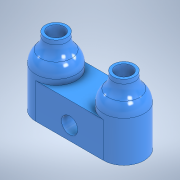
# Autodesk Inventor part: 4mm_Roller_Spacer_full
Saved by Autodesk Inventor 2021 (Build 250183000, 183)
## iProperties
Created: 2021-07-05
Part Number: 4mm_Roller_Spacer_full
Material: Generic
Document SubType Name: Modeling
Designer: Jorian Brusind
Density: 1 g/cm^3
Appearance: Cyan
Author: Jorian Brusind
Autodesk Inventor part; units mm, degrees
ref_plane "XZ Plane" through (0, 0, 0) normal (0, 1, 0) x (-1, 0, 0)
ref_plane "XY Plane" through (0, 0, 0) normal (0, 0, 1) x (1, 0, 0)
sketch "Sketch1" plane through (0, 0, 0) normal (0, 1, 0) x (-1, 0, 0)
  circle A0 centre (0, 0) radius 7.5
  circle A1 centre (0, 0) radius 3
  dimension "d0" = 15
  dimension "d1" = 6
  constraints: 2 centre point, 2 coincident
  measures "d0" diameter of A0
  measures "d1" diameter of A1
extrude "Extrusion1" add sketch "Sketch1" along normal blind 18
sketch "Sketch2" plane through (0, 18, 0) normal (0, 1, 0) x (1, 0, 0)
  circle A0 centre (0, 0) radius 3 projected
  circle A1 centre (0, 0) radius 2.75
  circle A2 centre (0, 0) radius 4
  dimension "d4" = 5.5
  dimension "d5" = 8
  constraints: 2 centre point, 2 coincident
  measures "d4" diameter of A1
  measures "d5" diameter of A2
extrude "Extrusion2" add sketch "Sketch2" along normal blind 7 contours A2
fillet "Fillet1" radius 6 1 edges at (-4, 18, 0)
fillet "Fillet2" radius 6 2 edges at (0, 18, -7.5) (0, 18, 7.5)
ref_plane "Work Plane1" through (12.5, 0, 0) normal (1, 0, 0) x (0, 1, 0)
mirror "Mirror1" about plane through (12.5, 0, 0) normal (1, 0, 0) of "Extrusion1", "Extrusion2", "Fillet1", "Fillet2"
sketch "Sketch3" plane through (0, 0, 0) normal (0, 1, 0) x (-1, 0, 0)
  circle A0 centre (-25, 0) radius 3 projected
  line L0 (-25, 0) -> (-25, 3)
  line L1 (-25, 0) -> (-25, -3)
  line L2 (0, 0) -> (0, -3)
  circle A1 centre (0, 0) radius 3 projected
  line L3 (0, 0) -> (0, 3)
  line L4 (-25, 3) -> (0, 3)
  line L5 (0, 3) -> (0, 7.5)
  line L6 (0, 7.5) -> (-25, 7.5)
  line L7 (-25, 7.5) -> (-25, 3)
  line L8 (-25, -3) -> (0, -3)
  line L9 (0, -3) -> (0, -7.5)
  line L10 (0, -7.5) -> (-25, -7.5)
  line L11 (-25, -7.5) -> (-25, -3)
  point P0 (0, -3)
  point P1 (0, 3)
  dimension "d11" = 25
  dimension "d12" = 4.5
  dimension "d13" = 25
  dimension "d14" = 4.5
  constraints: 24 end point, 4 parallel, 4 point on circle, 2 horizontal, 2 perpendicular, 2 point on line, 1 vertical
  measures "d11" distance of L6.end L5.end
  measures "d12" distance of L5.end L4.end
  measures "d13" distance of L9.end L10.end
  measures "d14" distance of L8.end L9.end
extrude "Extrusion3" add sketch "Sketch3" along normal blind 13 contours A0 L4 A1 L8 | L7 L6 L5 L4 | L8 L9 L10 L11
sketch "Sketch4" plane through (0, 0, 7.5) normal (0, 0, 1) x (1, 0, 0)
  line L0 (25, 13) -> (0, 13) projected
  circle A0 centre (12.5, 5) radius 3
  line L1 (0, 0) -> (25, 0) projected
  line L2 (0, 0) -> (0, 13) projected
  point P0 (25, 15)
  point P1 (0, 15)
  dimension "d18" = 6
  dimension "d21" = 5
  dimension "d22" = 12.5
  constraints: 1 centre point, 1 other
  measures "d18" diameter of A0
  measures "d21" distance from line of L1 A0.centre
  measures "d22" distance from line of L2 A0.centre
extrude "Extrusion4" cut sketch "Sketch4" against normal through all
body "Solid1"
